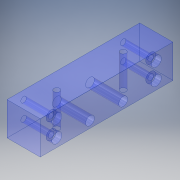
# Autodesk Inventor part: BackEndSlider
Saved by Autodesk Inventor 2019 (Build 230136000, 136)
## iProperties
Created: 2019-09-28
Part Number: BackEndSlider
Material: Generic
Document SubType Name: Modeling
Designer: james
Density: 1 g/cm^3
Appearance: Clear - Blue
Mass: 54.1046 g
Surface Area: 195.592 cm^2
Volume: 54.1046 cm^3
Author: james
Autodesk Inventor part; units mm, degrees
ref_plane "YZ Plane" through (0, 0, 0) normal (1, 0, 0) x (0, 1, 0)
ref_plane "XZ Plane" through (0, 0, 0) normal (0, 1, 0) x (-1, 0, 0)
ref_plane "XY Plane" through (0, 0, 0) normal (0, 0, 1) x (1, 0, 0)
sketch "Sketch1" plane through (0, 0, 0) normal (0, 0, 1) x (1, 0, 0)
  line L0 (-13.202, 13.202) -> (12.198, 13.202)
  line L1 (12.198, 13.202) -> (12.198, -12.198)
  line L2 (12.198, -12.198) -> (-13.202, -12.198)
  line L3 (-13.202, -12.198) -> (-13.202, 13.202)
  point P0 (0, 0)
  dimension "d0" = 25.4
  dimension "d1" = 25.4
  constraints: 8 end point, 2 parallel, 1 horizontal, 1 perpendicular
  measures "d0" distance of L1.end L2.end
  measures "d1" distance of L2.end L0.start
extrude "Extrusion1" add sketch "Sketch1" along normal blind 101.6
sketch "Sketch6" plane through (12.198, 13.202, 101.6) normal (1, 0, 0) x (0, 0, -1)
  line L0 (101.6, 0) -> (101.6, -25.4) projected
  line L1 (101.6, -25.4) -> (0, -25.4) projected
  line L2 (101.6, 0) -> (101.6, -25.4) projected
  line L3 (101.6, 0) -> (0, 0) projected
  line L4 (0, -25.4) -> (0, 0) projected
  line L5 (0, -25.4) -> (0, 0) projected
  point P0 (101.6, -13.202)
  point P1 (88.9, -6.35)
  point P2 (88.9, -19.05)
  point P3 (101.6, -19.05)
  point P4 (101.6, -6.35)
  point P5 (12.7, -6.35)
  point P6 (12.7, -19.05)
  point P7 (0, -19.05)
  point P8 (0, -6.35)
  dimension "d51" = 12.7
  dimension "d52" = 6.35
  dimension "d53" = 12.7
  dimension "d54" = 6.35
  dimension "d55" = 12.7
  dimension "d56" = 6.35
  dimension "d57" = 12.7
  dimension "d58" = 6.35
  measures "d51" distance from line of point (88.9, -19.05) L0
  measures "d52" distance from line of L1 point (88.9, -19.05)
  measures "d53" distance from line of L2 point (88.9, -6.35)
  measures "d54" distance from line of L3 point (88.9, -6.35)
  measures "d55" distance from line of L4 point (12.7, -19.05)
  measures "d56" distance from line of L1 point (12.7, -19.05)
  measures "d57" distance from line of L5 point (12.7, -6.35)
  measures "d58" distance from line of L3 point (12.7, -6.35)
hole "Hole5" at (12.198, 6.852, 12.7) at (12.198, -5.848, 12.7) at (12.198, 6.852, 88.9) at (12.198, -5.848, 88.9) direction (-1, 0, 0) diameter 4.318 end through all counterbore diameter 7.62 counterbore depth 4.318
sketch "Sketch9" plane through (-13.202, 13.202, 0) normal (0, 1, 0) x (1, 0, 0)
  line L0 (0, 0) -> (0, -101.6) projected
  line L1 (0, 0) -> (25.4, 0) projected
  line L2 (25.4, -101.6) -> (0, -101.6) projected
  point P0 (13.202, 0)
  point P1 (12.7, -25.4)
  point P2 (12.7, -76.2)
  dimension "d101" = 12.7
  dimension "d102" = 12.7
  dimension "d103" = 25.4
  dimension "d104" = 25.4
  measures "d101" distance from line of L0 point (12.7, -76.2)
  measures "d102" distance from line of L0 point (12.7, -25.4)
  measures "d103" distance from line of L1 point (12.7, -25.4)
  measures "d104" distance from line of L2 point (12.7, -76.2)
hole "Hole6" at (-0.502, 13.202, 25.4) at (-0.502, 13.202, 76.2) direction (0, -1, 0) diameter 4.4958 end through all clearance for "Flat Head Machine Screw (82)" size "#8" standard "Ansi Unified Screw Threads"
sketch "Sketch10" plane through (12.198, -12.198, 0) normal (1, 0, 0) x (0, 0, -1)
  line L0 (-101.6, 0) -> (-101.6, 25.4) projected
  line L1 (0, 25.4) -> (0, 0) projected
  line L2 (0, 0) -> (-101.6, 0) projected
  point P0 (0, 12.198)
  point P1 (-63.5, 5.08)
  point P2 (-38.1, 5.08)
  dimension "d112" = 38.1
  dimension "d113" = 38.1
  dimension "d114" = 5.08
  dimension "d115" = 5.08
  measures "d112" distance from line of L0 point (-63.5, 5.08)
  measures "d113" distance from line of L1 point (-38.1, 5.08)
  measures "d114" distance from line of L2 point (-38.1, 5.08)
  measures "d115" distance from line of L2 point (-63.5, 5.08)
hole "Hole7" at (12.198, -7.118, 63.5) at (12.198, -7.118, 38.1) direction (-1, 0, 0) diameter 6.7564 end through all clearance for "Flat Head Machine Screw (82)" size "1/4" standard "Ansi Unified Screw Threads"
body "Solid1"
